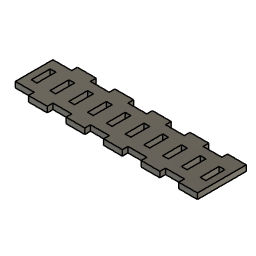
DiceHolder_SideWall_V7 v7 (Autodesk Fusion 360 design; units mm, degrees)
Autodesk Fusion 360 part; units mm, degrees
note: some values were not read from the file. Set by a fixed rule: which face or edge a step refers to.
sketch "Sketch1" plane through (0, 0, 0) normal (0, 0, 1) x (1, 0, 0)
  line L0 (-50, 15) -> (50, 15)
  line L1 (50, 15) -> (50, -15)
  line L2 (50, -15) -> (-50, -15)
  line L3 (-50, -15) -> (-50, 15)
  line L4 (-50, 15) -> (50, -15) construction
  line L5 (50, 15) -> (-50, -15) construction
  dimension "d1" = 100
  dimension "d2" = 30
  constraint horizontal L0
  constraint perpendicular L0 L1
  constraint parallel L0 L2
  constraint parallel L1 L3
  constraint coincident L4 origin
  constraint coincident L5 origin
  measures "d1" distance of L1.end L2.end
  measures "d2" distance of L0.end L1.end
extrude "Extrude1" add sketch "Sketch1" along normal blind 3
sketch "Sketch2" plane through (0, 0, 3) normal (0, 0, 1) x (-1, 0, 0)
  line L0 (50, 15) -> (-50, 15)
  line L1 (-50, 15) -> (-50, -15)
  line L2 (-50, -15) -> (50, -15)
  line L3 (50, -15) -> (50, 15)
  line L4 (50, 15) -> (40, 15)
  line L5 (40, 15) -> (40, 12)
  line L6 (40, 12) -> (50, 12)
  line L7 (50, 12) -> (50, 15)
  constraint horizontal L4
  constraint vertical L5
  constraint horizontal L6
  constraint vertical L7
  constraint coincident L0.start L3.end
extrude "Extrude2" cut sketch "Sketch2" against normal blind 9 contours L0 L3 L4 L5 L6 L7
sketch "Sketch3" plane through (0, 0, 3) normal (0, 0, 1) x (-1, 0, 0)
  line L0 (40, 12) -> (40, 15)
  line L1 (40, 15) -> (-50, 15)
  line L2 (-50, 15) -> (-50, -15)
  line L3 (-50, -15) -> (50, -15)
  line L4 (50, -15) -> (50, 12)
  line L5 (50, 12) -> (40, 12)
pattern_linear "R-Pattern1" count 5 spacing 20 along (1, 0, 0) count 2 spacing 27 along (0, 1, 0) of "Extrude2"
sketch "Sketch5" plane through (0, 0, 3) normal (0, 0, 1) x (-1, 0, 0)
  line L0 (-30, -12) -> (-30, -15)
  line L1 (-30, -15) -> (-20, -15)
  line L2 (-20, -15) -> (-20, -12)
  line L3 (-20, -12) -> (-10, -12)
  line L4 (-10, -12) -> (-10, -15)
  line L5 (-10, -15) -> (0, -15)
  line L6 (0, -15) -> (0, -12)
  line L7 (0, -12) -> (10, -12)
  line L8 (10, -12) -> (10, -15)
  line L9 (10, -15) -> (20, -15)
  line L10 (20, -15) -> (20, -12)
  line L11 (20, -12) -> (30, -12)
  line L12 (30, -12) -> (30, -15)
  line L13 (30, -15) -> (40, -15)
  line L14 (40, -15) -> (40, -12)
  line L15 (40, -12) -> (50, -12)
  line L16 (50, -12) -> (50, 12)
  line L17 (50, 12) -> (40, 12)
  line L18 (40, 12) -> (40, 15)
  line L19 (40, 15) -> (30, 15)
  line L20 (30, 15) -> (30, 12)
  line L21 (30, 12) -> (20, 12)
  line L22 (20, 12) -> (20, 15)
  line L23 (20, 15) -> (10, 15)
  line L24 (10, 15) -> (10, 12)
  line L25 (10, 12) -> (0, 12)
  line L26 (0, 12) -> (0, 15)
  line L27 (0, 15) -> (-10, 15)
  line L28 (-10, 15) -> (-10, 12)
  line L29 (-10, 12) -> (-20, 12)
  line L30 (-20, 12) -> (-20, 15)
  line L31 (-20, 15) -> (-30, 15)
  line L32 (-30, 15) -> (-30, 12)
  line L33 (-30, 12) -> (-40, 12)
  line L34 (-40, 12) -> (-40, 15)
  line L35 (-40, 15) -> (-50, 15)
  line L36 (-50, 15) -> (-50, -15)
  line L37 (-50, -15) -> (-40, -15)
  line L38 (-40, -15) -> (-40, -12)
  line L39 (-40, -12) -> (-30, -12)
  line L40 (43.5, 5) -> (46.5, 5)
  line L41 (46.5, 5) -> (46.5, -5)
  line L42 (46.5, -5) -> (43.5, -5)
  line L43 (43.5, -5) -> (43.5, 5)
  line L44 (43.5, 5) -> (46.5, -5) construction
  line L45 (46.5, 5) -> (43.5, -5) construction
  point P0 (45, 0)
  dimension "d13" = 3
  dimension "d14" = 10
  constraint horizontal L40
  constraint perpendicular L40 L41
  constraint parallel L40 L42
  constraint parallel L41 L43
  constraint coincident L44 P0
  constraint coincident L45 P0
  measures "d13" distance of L41.end L42.end
  measures "d14" distance of L40.end L41.end
extrude "Extrude4" cut sketch "Sketch5" against normal blind 9 contours L40 L41 L42 L43
pattern_linear "R-Pattern2" count 10 spacing 10 along (1, 0, 0) of "Extrude4"
extrude "Extrude5" cut 5 faces at (-46.6667, 12, 2) (-26.6667, 12, 2) (-6.6667, 12, 2) (13.3333, 12, 2) (33.3333, 12, 2) along direction (0, -1, 0) blind 2
extrude "Extrude6" cut 5 faces at (-33.3333, 15, 2) (-13.3333, 15, 2) (43.3333, 15, 1) (6.6667, 15, 2) (26.6667, 15, 2) along direction (0, -1, 0) blind 2
extrude "Extrude7" cut 5 faces at (-43.3333, -12, 2) (-23.3333, -12, 2) (-3.3333, -12, 2) (16.6667, -12, 2) (36.6667, -12, 2) along direction (0, 1, 0) blind 2
extrude "Extrude8" cut 5 faces at (46.6667, -15, 1) (-33.3333, -15, 1) (26.6667, -15, 1) (6.6667, -15, 1) (-13.3333, -15, 1) along direction (0, 1, 0) blind 2
extrude "Extrude3" [suppressed]
